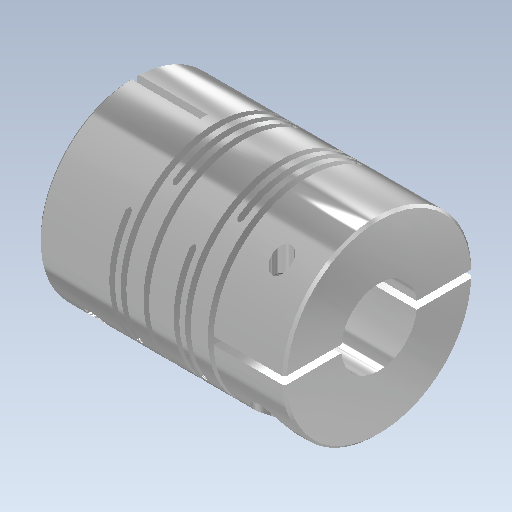
# Autodesk Inventor part: CPLSC20-8-8_b
Saved by Autodesk Inventor 2021 (Build 250183000, 183)
## iProperties
Category: PARTsolutions
Company: MISUMI
Part Number: CPLSC20-8-8_b
Material: アルミニウム 6061
Catalog Web Link: www.cadenas.de
Description: CPLCN, CPLSC_body-Couplings - Slit Clamping - Normal
Vendor: MISUMI
Document SubType Name: Modeling
Designer: partserver
Manufacturer: MISUMI
Mass: 14.5247 g
Surface Area: 64.1729 cm^2
Volume: 5.37953 cm^3
Density: 2.7 g/cm^3
Appearance: アルミニウム - フラット
PSOL_IDENT_0: {$CADENAS_DATA\23d-libs\misumi\metric\50_couplings\parts\cplcn.prj},211 {VTYP=3D},{NB=CPLSC20-8-8_b}
PSOL_IDENT_1: ,{LINA=CPLSC20-8-8},{NN=CPLCN, CPLSC_body},{DATE=30.03.2018 07:24:36},{GEOMDATE=03.12.2013 00:00:00}
PSOL_IDENT_2: ,{VERSION=},{LINEID=20},{WBVAR=MAT,ALT1,LDC,DD1,ALT2,RDC,DD2},{WBNUMERIC=LDC,RDC}  {NB=CPLSC20-8-8_b
PSOL_IDENT_3: },{LINA=CPLSC20-8-8},{KT=DUMMY},{PN=CPLSC20-8-8},{MAT=1},{ST=-},{AC=Hex Socket Head Cap Screw},{TYPE=
PSOL_IDENT_4: CPLSC},{D=20},{DDIA=20.000},{D1='5','5','6','6','6.35','6.35','8','8'},{ALT1=},{ALT1ALG=},{ALT1ALG2=
PSOL_IDENT_5: '', 'w/o LDC (Shaft Hole Diameter Left Shaft)', 'LDC'  , 'with LDC (Shaft Hole Diameter Left Shaft)'
PSOL_IDENT_6: },{LDC=0.000},{LDCALG=0},{LDCALG1=},{LDCMIN=5},{DLALT1=8},{DD1=8},{DD11=8},{DD1ALG1='5','5','6','6'
PSOL_IDENT_7: ,'6.35','6.35','8','8'},{DD1ALG2=8},{D2='8','8'},{ALT2=},{ALT2ALG=},{ALT2ALG1= '', 'w/o RDC (Shaft H
PSOL_IDENT_8: ole Diameter Right Shaft)', 'RDC'  , 'with RDC (Shaft Hole Diameter Right Shaft)' },{RDC=0.000},{RDC
PSOL_IDENT_9: ALG=[0]},{RDCALG1=},{DD2=8},{DD2ALG1='8','8'},{DD2ALG11='6','6','6.35','6.35','8','8'},{DD2ALG2=8},{
PSOL_IDENT_10: DL=8},{DR=8},{DD3=8.5},{L=26},{L1=26.000},{LL=7.5},{LL1=7.500},{M=2.5},{TSIMD=2.500},{TSIMIN=2.013},
PSOL_IDENT_11: {A=6.5},{A1=6.500},{F=3.75},{F1=3.750},{TSI=M2.5},{SC1=2.4000},{SC2=8.0000},{L2=6.800},{L3=0.600},{L
PSOL_IDENT_12: 4=15.600},{L5=0.800},{L6=1.200},{TSI1=4.900},{ALTALG2='','Select RDC'}
NB: CPLSC20-8-8_b
NN: CPLCN, CPLSC_body
NT: Couplings - Slit Clamping - Normal
NBSYN: $PN._b
LINA: CPLSC20-8-8
CATALOG: Misumi
PN: CPLSC20-8-8
MAT: Stainless Steel
ST: -
AC: Hex Socket Head Cap Screw
D: 20
ALT1: w/o LDC (Shaft Hole Diameter Left Shaft)
LDC: 0
DD1: 8
ALT2: w/o RDC (Shaft Hole Diameter Right Shaft)
RDC: 0
DD2: 8
L: 26
LL: 7.5
M: 2.5
A: 6.5
F: 3.75
SUPPLIER: MISUMI
ARTICLENO: CPLSC20-8-8_b
BOMINFO: CPLSC20-8-8
CREATOR: CADENAS GmbH
d19: 0.000 mm
d20: 0.000 mm
Title: CPLSC20-8-8
Author: Cadenas PARTsolutions
Comments: Couplings - Slit Clamping - Normal
Autodesk Inventor part; units mm, degrees
sketch "Sketch_1" plane through (0, 0, 0) normal (0, 0, 1) x (1, 0, 0)
  line L0 (26, 0) -> (0, 0)
  line L1 (0, 4) -> (7.5, 4)
  line L2 (7.5, 4) -> (7.5, 4.25)
  line L3 (7.5, 4.25) -> (18.5, 4.25)
  line L4 (18.5, 4.25) -> (18.5, 4)
  line L5 (18.5, 4) -> (26, 4)
  line L6 (26, 4) -> (26, 9.75)
  line L7 (26, 9.75) -> (25.75, 10)
  line L8 (25.75, 10) -> (0.25, 10)
  line L9 (0.25, 10) -> (0, 9.75)
  line L10 (0, 9.75) -> (0, 4)
  constraints: 22 end point
revolve "Revolution1" add sketch "Sketch_1" angle 360 about axis through (26, 0, 0) along (1, 0, 0)
sketch "Sketch_2" plane through (3.75, 0, 0) normal (1, 0, 0) x (0, 0, -1)
  line L0 (-10, -6.5) -> (10, -6.5)
  line L1 (10, -6.5) -> (10, -7.5065)
  line L2 (10, -7.5065) -> (0.6435, -7.5065)
  line L3 (0.6435, -7.5065) -> (0.4, -7.75)
  line L4 (0.4, -7.75) -> (-2.4, -7.75)
  line L5 (-2.4, -7.75) -> (-2.4, -8.95)
  line L6 (-2.4, -8.95) -> (-10, -8.95)
  line L7 (-10, -8.95) -> (-10, -6.5)
  line L8 (-10, -6.5) -> (10, -6.5)
  constraints: 18 end point
revolve "Revolution2" cut sketch "Sketch_2" angle 360 about axis through (3.75, -6.5, 10) along (0, 0, 1)
thread "Thread1" size "M2.5x0.45" class "6H" standard "ISO Metric profile" length 4.9565
sketch "Sketch_3" plane through (22.25, 0, 0) normal (1, 0, 0) x (0, 0, -1)
  line L0 (-6.5, 10) -> (-6.5, -10)
  line L1 (-6.5, -10) -> (-7.5065, -10)
  line L2 (-7.5065, -10) -> (-7.5065, -0.6435)
  line L3 (-7.5065, -0.6435) -> (-7.75, -0.4)
  line L4 (-7.75, -0.4) -> (-7.75, 2.4)
  line L5 (-7.75, 2.4) -> (-8.95, 2.4)
  line L6 (-8.95, 2.4) -> (-8.95, 10)
  line L7 (-8.95, 10) -> (-6.5, 10)
  line L8 (-6.5, 10) -> (-6.5, -10)
  constraints: 18 end point
revolve "Revolution3" cut sketch "Sketch_3" angle 360 about axis through (22.25, 10, 6.5) along (0, 1, 0)
thread "Thread2" size "M2.5x0.45" class "6H" standard "ISO Metric profile" length 4.9565
sketch "Sketch_4" plane through (0, 0, 0) normal (0, 0, 1) x (1, 0, 0)
  line L0 (7.5, 5.6) -> (7.5, -11.5)
  line L1 (7.5, -11.5) -> (14.9, -11.5)
  line L2 (14.9, -11.5) -> (14.9, 5.6)
  arc A0 (14.9, 5.6) -> (14.3, 5.6) centre (14.6, 5.6) ccw
  line L3 (14.3, 5.6) -> (14.3, -10.25)
  line L4 (14.3, -10.25) -> (8.1, -10.25)
  line L5 (8.1, -10.25) -> (8.1, 5.6)
  arc A1 (8.1, 5.6) -> (7.5, 5.6) centre (7.8, 5.6) ccw
  constraints: 12 end point, 4 point on circle, 2 centre point
extrude "Extrusion1" cut sketch "Sketch_4" along normal mid plane 21
sketch "Sketch_5" plane through (0, 0, 0) normal (0, 0, 1) x (1, 0, 0)
  arc A0 (8.7, -5.6) -> (9.3, -5.6) centre (9, -5.6) ccw
  line L0 (9.3, -5.6) -> (9.3, 10.25)
  line L1 (9.3, 10.25) -> (15.5, 10.25)
  line L2 (15.5, 10.25) -> (15.5, -5.6)
  arc A1 (15.5, -5.6) -> (16.1, -5.6) centre (15.8, -5.6) ccw
  line L3 (16.1, -5.6) -> (16.1, 11.5)
  line L4 (16.1, 11.5) -> (8.7, 11.5)
  line L5 (8.7, 11.5) -> (8.7, -5.6)
  constraints: 12 end point, 4 point on circle, 2 centre point
extrude "Extrusion2" cut sketch "Sketch_5" along normal mid plane 21
sketch "Sketch_6" plane through (0, 0, 0) normal (0, 1, 0) x (-1, 0, 0)
  line L0 (-11.1, -5.6) -> (-11.1, 11.5)
  line L1 (-11.1, 11.5) -> (-18.5, 11.5)
  line L2 (-18.5, 11.5) -> (-18.5, -5.6)
  arc A0 (-18.5, -5.6) -> (-17.9, -5.6) centre (-18.2, -5.6) ccw
  line L3 (-17.9, -5.6) -> (-17.9, 10.25)
  line L4 (-17.9, 10.25) -> (-11.7, 10.25)
  line L5 (-11.7, 10.25) -> (-11.7, -5.6)
  arc A1 (-11.7, -5.6) -> (-11.1, -5.6) centre (-11.4, -5.6) ccw
  constraints: 12 end point, 4 point on circle, 2 centre point
extrude "Extrusion3" cut sketch "Sketch_6" along normal mid plane 21
sketch "Sketch_7" plane through (0, 0, 0) normal (0, 1, 0) x (-1, 0, 0)
  arc A0 (-9.9, 5.6) -> (-10.5, 5.6) centre (-10.2, 5.6) ccw
  line L0 (-10.5, 5.6) -> (-10.5, -10.25)
  line L1 (-10.5, -10.25) -> (-16.7, -10.25)
  line L2 (-16.7, -10.25) -> (-16.7, 5.6)
  arc A1 (-16.7, 5.6) -> (-17.3, 5.6) centre (-17, 5.6) ccw
  line L3 (-17.3, 5.6) -> (-17.3, -11.5)
  line L4 (-17.3, -11.5) -> (-9.9, -11.5)
  line L5 (-9.9, -11.5) -> (-9.9, 5.6)
  constraints: 12 end point, 4 point on circle, 2 centre point
extrude "Extrusion4" cut sketch "Sketch_7" along normal mid plane 21
sketch "Sketch_8" plane through (0, 0, 0) normal (1, 0, 0) x (0, 1, 0)
  line L0 (10.25, 0.4) -> (-10.25, 0.4)
  line L1 (-10.25, 0.4) -> (-10.25, -0.4)
  line L2 (-10.25, -0.4) -> (10.25, -0.4)
  line L3 (10.25, -0.4) -> (10.25, 0.4)
  constraints: 8 end point
extrude "Extrusion5" cut sketch "Sketch_8" along normal blind 7.5
sketch "Sketch_9" plane through (26, 0, 0) normal (1, 0, 0) x (0, 0, -1)
  line L0 (-10.25, 0.4) -> (-10.25, -0.4)
  line L1 (-10.25, -0.4) -> (10.25, -0.4)
  line L2 (10.25, -0.4) -> (10.25, 0.4)
  line L3 (10.25, 0.4) -> (-10.25, 0.4)
  constraints: 8 end point
extrude "Extrusion6" cut sketch "Sketch_9" against normal blind 7.5
ref_plane "L1_XY" through (3.75, 6.5, 2.4) normal (0, 0, 1) x (1, 0, 0)
ref_plane "L1_YZ" through (3.75, 6.5, 2.4) normal (1, 0, 0) x (0, 1, 0)
ref_plane "L1_ZX" through (3.75, 6.5, 2.4) normal (0, 1, 0) x (0, 0, 1)
ref_plane "L2_XY" through (3.75, -6.5, 2.4) normal (0, 0, 1) x (1, 0, 0)
ref_plane "L2_YZ" through (3.75, -6.5, 2.4) normal (1, 0, 0) x (0, 1, 0)
ref_plane "L2_ZX" through (3.75, -6.5, 2.4) normal (0, 1, 0) x (0, 0, 1)
ref_plane "R1_XY" through (22.25, 2.4, -6.5) normal (0, 1, 0) x (1, 0, 0)
ref_plane "R1_YZ" through (22.25, 2.4, -6.5) normal (1, 0, 0) x (0, 0, -1)
ref_plane "R1_ZX" through (22.25, 2.4, -6.5) normal (0, 0, -1) x (0, 1, 0)
ref_plane "R2_XY" through (22.25, 2.4, 6.5) normal (0, 1, 0) x (1, 0, 0)
ref_plane "R2_YZ" through (22.25, 2.4, 6.5) normal (1, 0, 0) x (0, 0, -1)
ref_plane "R2_ZX" through (22.25, 2.4, 6.5) normal (0, 0, -1) x (0, 1, 0)
body "Solid1"
